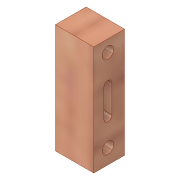
# Autodesk Inventor part: right side part
Saved by Autodesk Inventor 2019 (Build 230136000, 136)
## iProperties
Created: 2020-02-18
Part Number: right side part
Material: Wood (Oak)
Document SubType Name: Modeling
Designer: Admin
Density: 0.76 g/cm^3
Appearance: White Oak - Natural Medium Gloss
Author: Admin
Autodesk Inventor part; units mm, degrees
ref_plane "YZ Plane" through (0, 0, 0) normal (1, 0, 0) x (0, 1, 0)
ref_plane "XZ Plane" through (0, 0, 0) normal (0, 1, 0) x (-1, 0, 0)
ref_plane "XY Plane" through (0, 0, 0) normal (0, 0, 1) x (1, 0, 0)
sketch "Sketch1" plane through (0, 0, 0) normal (0, 0, 1) x (1, 0, 0)
  line L0 (0, 9.5048) -> (4.7524, 9.5048)
  line L1 (4.7524, 9.5048) -> (4.7524, -3.998)
  line L2 (4.7524, -3.998) -> (0, -3.998)
  line L3 (0, -3.998) -> (0, 9.5048)
  point P0 (0, 0)
  constraints: 8 end point, 2 parallel, 1 horizontal, 1 perpendicular
extrude "Extrusion1" add sketch "Sketch1" along normal blind 3.81
sketch "Sketch2" plane through (4.7524, -3.998, 0) normal (1, 0, 0) x (0, 0, -1)
  circle A0 centre (-2.0745, 12.0319) radius 0.7117
  circle A1 centre (-2.0745, 1.8482) radius 0.7112
  line L0 (-2.0745, 8.5619) -> (-2.0745, 5.1296) construction
  line L1 (-1.5841, 8.5619) -> (-1.5841, 5.1296)
  line L2 (-2.5648, 5.1296) -> (-2.5648, 8.5619)
  arc A2 (-1.5841, 8.5619) -> (-2.5648, 8.5619) centre (-2.0745, 8.5619) ccw
  arc A3 (-2.5648, 5.1296) -> (-1.5841, 5.1296) centre (-2.0745, 5.1296) ccw
  point P0 (0, 3.998)
  point P1 (-2.0745, 6.8457)
  constraints: 8 end point, 4 centre point, 4 point on circle, 4 tangent, 1 midpoint, 1 parallel, 1 vertical
extrude "Extrusion2" cut sketch "Sketch2" against normal blind 25.4
sketch "Sketch3" plane through (0, 0, 0) normal (0, 0, -1) x (-1, 0, 0)
  circle A0 centre (-2.5918, 2.6207) radius 0.0893
  point P0 (0, 0)
  constraints: 1 centre point
extrude "Extrusion3" cut sketch "Sketch3" against normal blind 3.048
body "Solid1"
